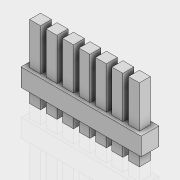
# Autodesk Inventor part: ЛЦМК.00002.00.00.00.00.01-01
Saved by Autodesk Inventor 2021.2 (Build 252289000, 289)
## iProperties
Created: 2025-10-22
Part Number: ЛЦМК.00002.00.00.00.00.01-01
Material: Типовые
Document SubType Name: Modeling
Designer: Захаров
Density: 1 g/cm^3
Appearance: По умолчанию
Author: Захаров
Autodesk Inventor part; units mm, degrees
ref_plane "YZ Plane" through (0, 0, 0) normal (1, 0, 0) x (0, 1, 0)
ref_plane "XZ Plane" through (0, 0, 0) normal (0, 1, 0) x (-1, 0, 0)
ref_plane "XY Plane" through (0, 0, 0) normal (0, 0, 1) x (1, 0, 0)
sketch "Эскиз1" plane through (0, 0, 0) normal (0, 0, 1) x (1, 0, 0)
  line L0 (8.75, -1.3) -> (-8.75, -1.3)
  line L1 (-8.75, -1.3) -> (-8.75, 1.3)
  line L2 (-8.75, 1.3) -> (8.75, 1.3)
  line L3 (8.75, 1.3) -> (8.75, -1.3)
  line L4 (8.75, -1.3) -> (-8.75, 1.3) construction
  line L5 (-8.75, -1.3) -> (8.75, 1.3) construction
  line L6 (-8, 7.4) -> (-6.4, 7.4)
  line L7 (-6.4, 7.4) -> (-6.4, 1.3)
  line L8 (-6.4, 1.3) -> (-8, 1.3)
  line L9 (-8, 1.3) -> (-8, 7.4)
  line L10 (-8, 1.3) -> (-7.2, 1.3)
  line L11 (-6.4, -3.2) -> (-8, -3.2)
  line L12 (-6.4, -1.3) -> (-6.4, -3.2)
  line L13 (-8, -3.2) -> (-8, -1.3)
  line L14 (-4, 7.4) -> (-4, 1.3)
  line L15 (-5.6, 1.3) -> (-5.6, 7.4)
  line L16 (-5.6, 7.4) -> (-4, 7.4)
  line L17 (-5.6, -3.2) -> (-5.6, -1.3)
  line L18 (-4, -1.3) -> (-4, -3.2)
  line L19 (-4, -3.2) -> (-5.6, -3.2)
  line L20 (-1.6, 7.4) -> (-1.6, 1.3)
  line L21 (-3.2, 1.3) -> (-3.2, 7.4)
  line L22 (-3.2, 7.4) -> (-1.6, 7.4)
  line L23 (-3.2, -3.2) -> (-3.2, -1.3)
  line L24 (-1.6, -1.3) -> (-1.6, -3.2)
  line L25 (-1.6, -3.2) -> (-3.2, -3.2)
  line L26 (0.8, 7.4) -> (0.8, 1.3)
  line L27 (-0.8, 1.3) -> (-0.8, 7.4)
  line L28 (-0.8, 7.4) -> (0.8, 7.4)
  line L29 (-0.8, -3.2) -> (-0.8, -1.3)
  line L30 (0.8, -1.3) -> (0.8, -3.2)
  line L31 (0.8, -3.2) -> (-0.8, -3.2)
  line L32 (3.2, 7.4) -> (3.2, 1.3)
  line L33 (1.6, 1.3) -> (1.6, 7.4)
  line L34 (1.6, 7.4) -> (3.2, 7.4)
  line L35 (1.6, -3.2) -> (1.6, -1.3)
  line L36 (3.2, -1.3) -> (3.2, -3.2)
  line L37 (3.2, -3.2) -> (1.6, -3.2)
  line L38 (5.6, 7.4) -> (5.6, 1.3)
  line L39 (4, 1.3) -> (4, 7.4)
  line L40 (4, 7.4) -> (5.6, 7.4)
  line L41 (4, -3.2) -> (4, -1.3)
  line L42 (5.6, -1.3) -> (5.6, -3.2)
  line L43 (5.6, -3.2) -> (4, -3.2)
  line L44 (8, 7.4) -> (8, 1.3)
  line L45 (6.4, 1.3) -> (6.4, 7.4)
  line L46 (6.4, 7.4) -> (8, 7.4)
  line L47 (6.4, -3.2) -> (6.4, -1.3)
  line L48 (8, -1.3) -> (8, -3.2)
  line L49 (8, -3.2) -> (6.4, -3.2)
  point P0 (0, 0)
  point P1 (8, -1.3)
  point P2 (6.4, -1.3)
  point P3 (5.6, -1.3)
  point P4 (4, -1.3)
  point P5 (3.2, -1.3)
  point P6 (1.6, -1.3)
  point P7 (0.8, -1.3)
  point P8 (-0.8, -1.3)
  point P9 (-1.6, -1.3)
  point P10 (-3.2, -1.3)
  point P11 (-4, -1.3)
  point P12 (-5.6, -1.3)
  point P13 (-5.6, 1.3)
  point P14 (-4, 1.3)
  point P15 (-3.2, 1.3)
  point P16 (-1.6, 1.3)
  point P17 (-0.8, 1.3)
  point P18 (0.8, 1.3)
  point P19 (6.4, 1.3)
  point P20 (8, 1.3)
  point P21 (1.6, 1.3)
  point P22 (3.2, 1.3)
  point P23 (4, 1.3)
  point P24 (5.6, 1.3)
  point P25 (-6.4, 1.3)
  dimension "d0" = 17.5
  dimension "d1" = 2.6
  dimension "d3" = 8.7
  dimension "d7" = 4.5
  dimension "d8" = 0.75
  dimension "d9" = 1.6
  dimension "d12" = 2.4
  constraints: 100 end point, 6 parallel, 4 horizontal, 3 midpoint, 3 perpendicular, 3 point on line, 2 collinear, 83 other
  measures "d0" distance of L1.end L2.end
  measures "d1" distance of L0.end L1.end
  measures "d3" distance between parallel lines of L6 L0
  measures "d7" distance between parallel lines of L2 L11
  measures "d8" horizontal distance of L0.end L11.end
  measures "d9" distance of L6.start L6.end
  measures "d12" distance of L6.end L14.start
extrude "Выдавливание1" add sketch "Эскиз1" against normal mid plane 2.6 contours L0 L1 L2 L3
extrude "Выдавливание2" add sketch "Эскиз1" along normal mid plane 1.6 contours L48 L49 L47 L0 | L2 L45 L46 L44 | L42 L43 L41 L0 | L2 L39 L40 L38 | L36 L37 L35 L0 | L2 L33 L34 L32 | L30 L31 L29 L0 | L2 L27 L28 L26 | L24 L25 L23 L0 | L2 L21 L22 L20 | L18 L19 L17 L0 | L2 L15 L16 L14 | L12 L11 L13 L0 | L2 L9 L6 L7
